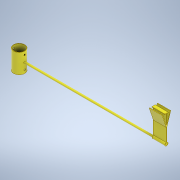
# Autodesk Inventor part: LDR
Saved by Autodesk Inventor 2022 (Build 260153000, 153)
## iProperties
Created: 2021-10-04
Part Number: LDR
Material: Genérico
Document SubType Name: Modeling
Designer: Alison
Density: 1 g/cm^3
Appearance: Ouro - Metal
Author: Alison
Autodesk Inventor part; units mm, degrees
ref_plane "YZ Plane" through (0, 0, 0) normal (1, 0, 0) x (0, 1, 0)
ref_plane "XZ Plane" through (0, 0, 0) normal (0, 1, 0) x (-1, 0, 0)
ref_plane "XY Plane" through (0, 0, 0) normal (0, 0, 1) x (1, 0, 0)
sketch "Esboço1" plane through (0, 0, 0) normal (0, 1, 0) x (-1, 0, 0)
  circle A0 centre (0, 0) radius 16
  circle A1 centre (0, 0) radius 17.5
  dimension "d0" = 32
  dimension "d1" = 35
  constraints: 2 centre point, 2 coincident
  measures "d0" diameter of A0
  measures "d1" diameter of A1
extrude "Extrusão1" add sketch "Esboço1" along normal mid plane 60
sketch "Esboço2" plane through (0, 0, 0) normal (0, 1, 0) x (-1, 0, 0)
  circle A0 centre (0, 0) radius 17.5 projected
  line L0 (-17.5, 0) -> (-417.5, 0)
  line L1 (-417.5, 0) -> (-417.5, 3)
  circle A1 centre (0, 0) radius 9.5
  line L2 (-26.4835, 0) -> (-26.4835, 3)
  line L3 (-17.2409, 3) -> (-417.5, 3)
  point P0 (-15.8635, 7.3891)
  dimension "d4" = 400
  dimension "d5" = 3
  dimension "d6" = 19
  dimension "d60" = 3
  constraints: 8 end point, 3 point on circle, 2 vertical, 1 centre point, 1 coincident, 1 horizontal, 1 parallel, 1 point on line
  measures "d4" distance of L0.start L0.end
  measures "d5" distance of L0.end L1.end
  measures "d6" diameter of A1
  measures "d60" distance of L2.start L2.end
revolve "Revolução1" add sketch "Esboço2" angle 360 about axis through (17.5, 0, 0) along (1, 0, 0) contours A0 L0 L2 L3 | L2 L0 L1 L3
sketch "Esboço3" plane through (0, 0, 0) normal (0, 1, 0) x (-1, 0, 0)
  line L0 (-417.5, -3) -> (-417.5, 3) projected
  line L1 (-417.5, 0) -> (-417.5, 15)
  line L2 (-417.5, 15) -> (-417.5, -15)
  line L3 (-417.5, -15) -> (-457.5, -15)
  line L4 (-457.5, -15) -> (-457.5, 15)
  line L5 (-457.5, 15) -> (-417.5, 15)
  point P0 (0, 0)
  dimension "d8" = 15
  dimension "d9" = 30
  dimension "d10" = 40
  constraints: 10 end point, 3 perpendicular, 1 collinear, 1 midpoint, 1 point on line
  measures "d8" distance of L1.start L1.end
  measures "d9" distance of L1.end L2.end
  measures "d10" distance of L2.end L3.end
extrude "Extrusão2" add sketch "Esboço3" along normal mid plane 170
sketch "Esboço5" plane through (457.5, -85, -15) normal (1, 0, 0) x (0, 0, -1)
  circle A0 centre (-15, 85) radius 4
  circle A1 centre (-15, 85) radius 3 projected
  line L0 (-16.25, 88.0318) -> (-14.25, 88.0318)
  line L1 (-14.25, 88.0318) -> (-14.25, 87.9047)
  line L2 (-14.25, 87.9047) -> (0, 87.9047)
  line L3 (0, 0) -> (0, 170) projected
  line L4 (-15.75, 87.9047) -> (-30, 87.9047)
  line L5 (-30, 170) -> (-30, 0) projected
  line L6 (-30, 87.9047) -> (-30, 0)
  line L7 (0, 0) -> (-30, 0) projected
  line L8 (-30, 0) -> (0, 0)
  line L9 (0, 0) -> (0, 87.9047)
  circle A2 centre (-15, 85) radius 5
  line L10 (-15.9946, 130.4066) -> (-13.9946, 130.4094)
  line L11 (-13.9946, 130.4094) -> (-14.0909, 89.9167)
  line L12 (-15.9946, 130.4066) -> (-28.3553, 168.4488)
  line L13 (-15.9946, 130.4066) -> (24.0054, 130.4066) construction
  line L14 (-13.9946, 130.4094) -> (-1.6339, 168.4517)
  line L15 (-13.9946, 130.4094) -> (26.0054, 130.4094) construction
  line L16 (-18.099, 136.8832) -> (-16.1969, 137.5013)
  line L17 (-25.4193, 159.413) -> (-23.5172, 160.031)
  line L18 (-4.4713, 159.7191) -> (-6.3734, 160.3371)
  line L19 (-10.3922, 141.4965) -> (-12.2943, 142.1146)
  line L20 (-28.3553, 168.4488) -> (-26.2523, 168.4488)
  line L21 (-1.6339, 168.4517) -> (-3.7368, 168.4517)
  line L22 (-15.0524, 134.2763) -> (-15.0666, 134.2336)
  line L23 (-15.9946, 168.4488) -> (-13.9946, 168.4488)
  line L24 (-15.9946, 89.9001) -> (-15.9946, 130.4066)
  line L25 (-15.9946, 136.8787) -> (-15.9946, 168.4488)
  line L26 (-13.9946, 168.4488) -> (-13.9946, 136.8787)
  line L27 (-15.9946, 136.8787) -> (-26.2523, 168.4488)
  line L28 (-13.9946, 136.8787) -> (-3.7368, 168.4517)
  line L29 (-15.9946, 168.4488) -> (-19.9946, 168.4488)
  line L30 (-19.9946, 168.4488) -> (-9.9946, 168.4488)
  line L31 (-9.9946, 168.4488) -> (-9.9946, 166.4488)
  line L32 (-9.9946, 166.4488) -> (-19.9946, 166.4488)
  line L33 (-19.9946, 166.4488) -> (-19.9946, 168.4488)
  line L34 (-15.9946, 168.4488) -> (-15.9946, 156.4488)
  line L35 (-15.9946, 156.4488) -> (-18.9946, 156.4488)
  line L36 (-18.9946, 156.4488) -> (-18.9946, 146.4488)
  line L37 (-18.9946, 146.4488) -> (-15.9946, 146.4488)
  line L38 (-13.9946, 156.4488) -> (-10.9946, 156.4488)
  line L39 (-10.9946, 156.4488) -> (-10.9946, 146.4488)
  line L40 (-10.9946, 146.4488) -> (-13.9946, 146.4488)
  line L41 (-30, 170) -> (0, 170) projected
  line L42 (-30, 170) -> (-30, 0)
  line L43 (0, 0) -> (0, 170) projected
  line L44 (0, 0) -> (-30, 0)
  line L45 (0, 0) -> (0, 170)
  line L46 (-30, 170) -> (0, 170)
  point P0 (-15, 85)
  point P1 (-15.9946, 166.4488)
  point P2 (-13.9946, 166.4488)
  dimension "d15" = 10
  dimension "d17" = 2
  dimension "d19" = 40
  dimension "d20" = 108
  dimension "d21" = 40
  dimension "d22" = 72
  dimension "d23" = 2
  dimension "d24" = 2
  dimension "d25" = 2
  dimension "d26" = 2
  dimension "d29" = 36
  dimension "d31" = 2
  dimension "d34" = 4
  dimension "d35" = 10
  dimension "d36" = 2
  dimension "d37" = 12
  dimension "d38" = 3
  dimension "d39" = 10
  dimension "d40" = 3
  dimension "d42" = 10
  constraints: 84 end point, 13 perpendicular, 13 point on line, 6 horizontal, 4 point on circle, 3 collinear, 3 vertical, 2 centre point, 2 coincident, 2 equal length, 2 parallel
  measures "d15" diameter of A2
  measures "d17" distance of L10.start L10.end
  measures "d19" distance of L10.start L12.end
  measures "d20" angle of L13 L12
  measures "d21" distance of L10.end L14.end
  measures "d22" angle of L15 L14
  measures "d23" distance of L16.start L16.end
  measures "d24" distance of L17.start L17.end
  measures "d25" distance of L18.start L18.end
  measures "d26" distance of L19.start L19.end
  measures "d29" distance of L21.end L22.start
  measures "d31" distance of L23.start L23.end
  measures "d34" distance of L23.start L29.end
  measures "d35" distance of L29.end L30.end
  measures "d36" distance of L30.end L31.end
  measures "d37" distance of L23.start L34.end
  measures "d38" distance of L34.end L35.end
  measures "d39" distance of L35.end L36.end
  measures "d40" distance of L38.start L38.end
  measures "d42" distance of L38.end L39.end
extrude "Extrusão3" cut sketch "Esboço5" against normal blind 170 contours A2 L11 L14 L21 L28 L26 L40 L39 L38 L32 L31 L30 L23 L29 L33 L25 L35 L36 L37 L27 L20 L12 L24 L4 L5 L41 L3 L2 | L2 L3 L7 L5 L4 A2
sketch "Esboço6" plane through (457.5, 4.9001, 0.9946) normal (1, 0, 0) x (0, 0, -1)
  circle A0 centre (0.9946, -4.9001) radius 3
  dimension "d61" = 6
  constraints: 1 centre point, 1 coincident
  measures "d61" diameter of A0
extrude "Extrusão4" cut sketch "Esboço6" against normal blind 0.01
sketch "Esboço7" plane through (457.5, 4.9001, 0.9946) normal (1, 0, 0) x (0, 0, -1)
  line L0 (0, 66.5487) -> (-3, 66.5487) projected
  line L1 (-3, 56.5487) -> (0, 56.5487) projected
  line L2 (0, 66.5487) -> (0, 56.5487)
  line L3 (0, 56.5487) -> (-3, 56.5487)
  line L4 (-3, 66.5487) -> (-3, 56.5487) projected
  line L5 (-3, 56.5487) -> (-3, 66.5487)
  line L6 (-3, 66.5487) -> (0, 66.5487)
  line L7 (2, 56.5487) -> (5, 56.5487) projected
  line L8 (2, 56.5487) -> (5, 56.5487)
  line L9 (2, 66.5487) -> (5, 66.5487) projected
  line L10 (5, 56.5487) -> (5, 66.5487)
  line L11 (5, 66.5487) -> (2, 66.5487)
  line L12 (2, 66.5487) -> (2, 56.5487)
  point P0 (0.9946, -4.9001)
  constraints: 16 end point, 5 perpendicular, 2 collinear, 1 vertical
extrude "Extrusão5" cut sketch "Esboço7" against normal blind 10
sketch "Esboço8" plane through (417.5, 4.9001, 0.9946) normal (-1, 0, 0) x (0, 0, 1)
  line L0 (-2, 76.5487) -> (-2, 66.5487) projected
  line L1 (-2, 56.5487) -> (-2, 46.9786) projected
  line L2 (-2, 66.5487) -> (-2, 56.5487)
  line L3 (-5, 56.5487) -> (-2, 56.5487) projected
  line L4 (-2, 56.5487) -> (-5, 56.5487)
  line L5 (-5, 56.5487) -> (-5, 66.5487)
  line L6 (-5, 66.5487) -> (-2, 66.5487)
  line L7 (3, 66.5487) -> (0, 66.5487) projected
  line L8 (0, 66.5487) -> (3, 66.5487)
  line L9 (3, 66.5487) -> (3, 56.5487)
  line L10 (0, 46.9786) -> (0, 56.5487) projected
  line L11 (3, 56.5487) -> (0, 56.5487)
  line L12 (0, 56.5487) -> (0, 66.5487)
  line L13 (0, 76.5487) -> (0, 46.9786) projected
  point P0 (-0.9946, -4.9001)
  constraints: 16 end point, 5 perpendicular, 2 collinear, 2 point on line, 1 vertical
extrude "Extrusão6" cut sketch "Esboço8" against normal blind 15
fillet "Arredondamento1" radius 5 4 edges at (447.5, 71.4488, 2.4946) (447.5, 61.4488, 2.4946) (447.5, 61.4488, -2.5054) (447.5, 71.4488, -2.5054)
sketch "Esboço9" plane through (0, 0, 0) normal (1, 0, 0) x (0, 1, 0)
  line L0 (30, -17.5) -> (30, 17.5) projected
  line L1 (30, 0) -> (20, 0)
  line L2 (-30, -16) -> (-30, 16) projected
  line L3 (-30, 0) -> (-20, 0)
  circle A0 centre (20, 0) radius 2.5
  circle A1 centre (-20, 0) radius 2.5
  point P0 (0, 0)
  dimension "d52" = 10
  dimension "d53" = 10
  dimension "d56" = 5
  dimension "d57" = 5
  constraints: 4 end point, 2 centre point, 2 coincident, 2 horizontal, 2 midpoint
  measures "d52" distance of L1.start L1.end
  measures "d53" distance of L3.start L3.end
  measures "d56" diameter of A0
  measures "d57" diameter of A1
extrude "Extrusão7" cut sketch "Esboço9" along normal mid plane 150
